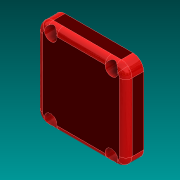
# Autodesk Inventor part: gearbox v2
Saved by Autodesk Inventor 2020 (Build 240168000, 168)
## iProperties
Created: 2020-05-25
Part Number: gearbox v2
Material: Generic
Document SubType Name: Modeling
Designer: stefa
Density: 1 g/cm^3
Appearance: Smooth - Red
Author: stefa
Autodesk Inventor part; units mm, degrees
ref_plane "YZ Plane" through (0, 0, 0) normal (1, 0, 0) x (0, 1, 0)
ref_plane "XZ Plane" through (0, 0, 0) normal (0, 1, 0) x (-1, 0, 0)
ref_plane "XY Plane" through (0, 0, 0) normal (0, 0, 1) x (1, 0, 0)
sketch "Sketch1" plane through (0, 0, 0) normal (0, 0, 1) x (1, 0, 0)
  line L0 (-25, -25) -> (25, -25)
  line L1 (25, -25) -> (25, 25)
  line L2 (25, 25) -> (-25, 25)
  line L3 (-25, 25) -> (-25, -25)
  line L4 (-25, -25) -> (25, 25) construction
  line L5 (25, -25) -> (-25, 25) construction
  line L6 (-15, 15) -> (15, 15)
  line L7 (15, 15) -> (15, -15)
  line L8 (15, -15) -> (-15, -15)
  line L9 (-15, -15) -> (-15, 15)
  circle A0 centre (0, 0) radius 11
  circle A1 centre (0, 0) radius 4.5
  circle A2 centre (-17, 21) radius 2
  circle A3 centre (17, 21) radius 2
  circle A4 centre (-17, -21) radius 2
  circle A5 centre (17, -21) radius 2
  dimension "d0" = 50
  dimension "d1" = 50
  dimension "d2" = 10
  dimension "d3" = 22
  dimension "d4" = 9
  dimension "d19" = 4
  dimension "d20" = 4
  dimension "d23" = 34
  dimension "d26" = 42
  dimension "d32" = 8
  constraints: 20 end point, 6 centre point, 4 parallel, 2 coincident, 2 horizontal, 2 midpoint, 2 perpendicular, 1 vertical, 9 other
  measures "d0" distance of L2.end L1.end
  measures "d1" distance of L1.end L0.end
  measures "d2" distance between parallel lines of L2 L6
  measures "d3" diameter of A0
  measures "d4" diameter of A1
  measures "d19" diameter of A2
  measures "d20" distance from line of L2 A2.centre
  measures "d23" distance of A2.centre A3.centre
  measures "d26" distance of A2.centre A4.centre
  measures "d32" distance from line of L3 A2.centre
extrude "Extrusion1" add sketch "Sketch1" along normal blind 10 contours L3 L2 L1 L0 | L6 L7 L8 L9 | A0 | A1 | A2 | A3 | A4 | A5
extrude "Extrusion3" cut sketch "Sketch1" along normal blind 7 contours A0
extrude "Extrusion4" cut sketch "Sketch1" along normal through all contours A2 | A3 | A4 | A5
extrude "Extrusion7" cut sketch "Sketch1" along normal blind 9 contours A1
fillet "Fillet1" radius 6 4 edges at (-25, 25, 5) (-25, -25, 5) (25, 25, 5) (25, -25, 5)
sketch "Sketch4" plane through (0, 0, 10) normal (0, 0, 1) x (1, 0, 0)
  circle A0 centre (0, 0) radius 11 projected
  arc A1 (19, -25) -> (25, -19) centre (19, -19) ccw projected
  line L0 (25, -19) -> (25, 19) projected
  arc A2 (25, 19) -> (19, 25) centre (19, 19) ccw projected
  line L1 (19, 25) -> (-19, 25) projected
  arc A3 (-19, 25) -> (-25, 19) centre (-19, 19) ccw projected
  line L2 (-25, 19) -> (-25, -19) projected
  arc A4 (-25, -19) -> (-19, -25) centre (-19, -19) ccw projected
  line L3 (-19, -25) -> (19, -25) projected
  circle A5 centre (17, -21) radius 2 projected
  circle A6 centre (-17, -21) radius 2 projected
  circle A7 centre (17, 21) radius 2 projected
  circle A8 centre (-17, 21) radius 2 projected
  circle A9 centre (17, -21) radius 3.55
  circle A10 centre (-17, -21) radius 2 projected
  circle A11 centre (-17, -21) radius 3.55
  circle A12 centre (-17, 21) radius 3.55
  circle A13 centre (17, 21) radius 3.55
  dimension "d46" = 7.1
  constraints: 4 centre point, 4 coincident, 3 equal radius
  measures "d46" diameter of A9
extrude "Extrusion9" cut sketch "Sketch4" against normal blind 7 contours A6 | A9 | A11 | A12 | A13
fillet "Fillet3" radius 3.5 8 edges at (-23.2426, -23.2426, 10) (0, -25, 10) (23.2426, -23.2426, 10) (25, 0, 10) (23.2426, 23.2426, 10) (0, 25, 10) (-23.2426, 23.2426, 10) (-25, 0, 10)
equation "\"d23\" = d1 - 2 * d32"
equation "\"d26\" = d0 - 2 * d20"
body "Solid1"
